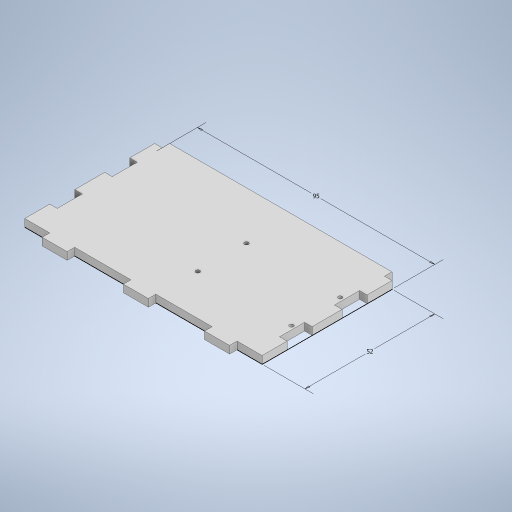
# Autodesk Inventor part: Parede_lateral_3
Saved by Autodesk Inventor 2024 (Build 280153000, 153)
## iProperties
Created: 2023-11-29
Part Number: Parede_lateral_3
Material: Genérico
Document SubType Name: Modeling
Designer: caiot
Density: 1 g/cm^3
Appearance: Padrão
Author: caiot
Autodesk Inventor part; units mm, degrees
ref_plane "YZ Plane" through (0, 0, 0) normal (1, 0, 0) x (0, 1, 0)
ref_plane "XZ Plane" through (0, 0, 0) normal (0, 1, 0) x (-1, 0, 0)
ref_plane "XY Plane" through (0, 0, 0) normal (0, 0, 1) x (1, 0, 0)
sketch "Parede_lateral_1" plane through (0, 0, 0) normal (0, 1, 0) x (-1, 0, 0)
  line L0 (0, 0) -> (-95, 0)
  line L1 (-95, 0) -> (-95, -52)
  line L2 (-95, -52) -> (0, -52)
  line L3 (0, -52) -> (0, 0)
  dimension "d0" = 95
  dimension "d1" = 52
  constraints: 8 end point, 2 parallel, 1 horizontal, 1 perpendicular
  measures "d0" distance of L2.end L1.end
  measures "d1" distance of L1.end L0.end
extrude "Extrusão1" add sketch "Parede_lateral_1" along normal blind 3
sketch "Esboço4" plane through (0, 3, 0) normal (0, 1, 0) x (1, 0, 0)
  line L0 (0, 52) -> (0, 0) projected
  line L1 (0, 42) -> (3, 42)
  line L2 (3, 42) -> (3, 32)
  line L3 (3, 32) -> (0, 32)
  line L4 (0, 32) -> (0, 42)
  line L5 (0, 20) -> (3, 20)
  line L6 (3, 20) -> (3, 10)
  line L7 (3, 10) -> (0, 10)
  line L8 (0, 10) -> (0, 20)
  line L9 (95, 0) -> (95, 52) projected
  line L10 (0, 0) -> (95, 0) projected
  line L11 (95, 42) -> (92, 42)
  line L12 (92, 42) -> (92, 32)
  line L13 (92, 32) -> (95, 32)
  line L14 (95, 32) -> (95, 42)
  line L15 (95, 20) -> (92, 20)
  line L16 (92, 20) -> (92, 10)
  line L17 (92, 10) -> (95, 10)
  line L18 (95, 10) -> (95, 20)
  line L19 (10, 0) -> (20, 0)
  line L20 (20, 0) -> (20, -3)
  line L21 (20, -3) -> (10, -3)
  line L22 (10, -3) -> (10, 0)
  line L23 (42.5, 0) -> (52.5, 0)
  line L24 (52.5, 0) -> (52.5, -3)
  line L25 (52.5, -3) -> (42.5, -3)
  line L26 (42.5, -3) -> (42.5, 0)
  line L27 (75, 0) -> (85, 0)
  line L28 (85, 0) -> (85, -3)
  line L29 (85, -3) -> (75, -3)
  line L30 (75, -3) -> (75, 0)
  point P0 (1.5, 42)
  point P1 (1.5, 10)
  dimension "d37" = 3
  dimension "d38" = 10
  dimension "d39" = 3
  dimension "d40" = 10
  dimension "d46" = 10
  dimension "d47" = 3
  dimension "d49" = 3
  constraints: 56 end point, 14 parallel, 10 point on line, 7 horizontal, 7 perpendicular, 2 midpoint
  measures "d37" distance of L2.end L3.end
  measures "d38" distance of L1.end L2.end
  measures "d39" distance of L6.end L7.end
  measures "d40" distance of L5.end L6.end
  measures "d46" distance from line of point (1.5, 10) L10
  measures "d47" distance of L13.end L12.end
  measures "d49" distance of L19.end L20.end
extrude "Extrusão4" add sketch "Esboço4" against normal blind 3 contours L10 L28 L29 L30 | L10 L24 L25 L26 | L10 L20 L21 L22
sketch "Esboço5" plane through (0, 3, 0) normal (0, 1, 0) x (1, 0, 0)
  line L0 (0, 52) -> (0, 0) projected
  line L1 (0, 10) -> (3, 10)
  line L2 (3, 10) -> (3, 20)
  line L3 (3, 20) -> (0, 20)
  line L4 (0, 20) -> (0, 10)
  line L5 (0, 32) -> (3, 32)
  line L6 (3, 32) -> (3, 42)
  line L7 (3, 42) -> (0, 42)
  line L8 (0, 42) -> (0, 32)
  line L9 (95, 52) -> (0, 52) projected
  line L10 (0, 0) -> (10, 0) projected
  line L11 (95, 0) -> (95, 52) projected
  line L12 (95, 42) -> (92, 42)
  line L13 (92, 42) -> (92, 32)
  line L14 (92, 32) -> (95, 32)
  line L15 (95, 32) -> (95, 42)
  line L16 (95, 20) -> (92, 20)
  line L17 (92, 20) -> (92, 10)
  line L18 (92, 10) -> (95, 10)
  line L19 (95, 10) -> (95, 20)
  point P0 (10, 52)
  point P1 (1.5, 42)
  point P2 (1.5, 10)
  dimension "d52" = 3
  dimension "d53" = 10
  dimension "d54" = 3
  dimension "d55" = 10
  dimension "d56" = 10
  dimension "d57" = 10
  dimension "d58" = 3
  constraints: 32 end point, 8 parallel, 5 point on line, 4 horizontal, 4 perpendicular, 2 midpoint
  measures "d52" distance of L3.end L2.end
  measures "d53" distance of L2.end L1.end
  measures "d54" distance of L7.end L6.end
  measures "d55" distance of L6.end L5.end
  measures "d56" distance from line of L9 point (1.5, 42)
  measures "d57" distance from line of L10 point (1.5, 10)
  measures "d58" distance of L14.end L13.end
extrude "Extrusão5" cut sketch "Esboço5" against normal blind 3
sketch "Esboço17" plane through (0, 3, 0) normal (0, 1, 0) x (1, 0, 0)
  line L0 (53, 35.75) -> (90.5, 35.75)
  line L1 (90.5, 35.75) -> (90.5, 16.25)
  line L2 (90.5, 16.25) -> (53, 16.25)
  line L3 (53, 16.25) -> (53, 35.75)
  line L4 (95, 53) -> (0, 53) projected
  line L5 (92, 32) -> (92, 42) projected
  circle A0 centre (90.5, 35.75) radius 0.8
  circle A1 centre (90.5, 16.25) radius 0.8
  circle A2 centre (53, 16.25) radius 0.8
  circle A3 centre (53, 35.75) radius 0.8
  line L6 (85, 0) -> (95, 0) projected
  line L7 (95, 32) -> (92, 32) projected
  line L8 (92, 20) -> (95, 20) projected
  line L9 (52.5, 0) -> (75, 0) projected
  line L10 (95, 52) -> (0, 52) projected
  point P0 (0, 0)
  point P1 (90.5, 26)
  point P2 (93.5, 32)
  point P3 (93.5, 20)
  dimension "d130" = 37.5
  dimension "d131" = 19.5
  dimension "d133" = 1.5
  dimension "d134" = 1.6
  dimension "d135" = 1.6
  dimension "d136" = 1.6
  dimension "d137" = 1.6
  dimension "d143" = 3.75
  dimension "d144" = 3.75
  dimension "d146" = 16.25
  constraints: 8 end point, 4 centre point, 4 coincident, 3 midpoint, 2 parallel, 1 horizontal, 1 perpendicular
  measures "d130" distance of L1.end L2.end
  measures "d131" distance of L0.end L1.end
  measures "d133" distance from line of L5 point (90.5, 26)
  measures "d134" diameter of A0
  measures "d135" diameter of A1
  measures "d136" diameter of A2
  measures "d137" diameter of A3
  measures "d143" vertical distance of point (93.5, 32) L0.end
  measures "d144" vertical distance of point (93.5, 20) L1.end
  measures "d146" distance from line of L0.end L10
extrude "Extrusão14" cut sketch "Esboço17" against normal blind 3 contours L3 A3 L0 | L0 A3 L3 | A0 L1 L0 | L0 L1 A0 | A2 L2 L3 | L3 L2 A2 | A1 L2 L1 | L1 L2 A1
sketch "Esboço18" plane through (0, 0, 0) normal (0, -1, 0) x (1, 0, 0)
  line L0 (0, -42) -> (3, -42) projected
  line L1 (92, -42) -> (92, -32) projected
  line L2 (92, -42) -> (92, -52)
  line L3 (3, -42) -> (3, -52)
  line L4 (95, -52) -> (0, -52) projected
  line L5 (3, -52) -> (92, -52)
  line L6 (92, -52) -> (92, -55)
  line L7 (92, -55) -> (3, -55)
  line L8 (3, -55) -> (3, -52)
  point P0 (0, 0)
  dimension "d150" = 3
  constraints: 12 end point, 2 parallel, 2 vertical, 1 horizontal, 1 perpendicular, 1 point on line
  measures "d150" distance of L5.end L6.end
extrude "Extrusão15" add sketch "Esboço18" against normal blind 3
equation "\"d146\" = -0.5 * d131 + 0.5 * d1"
